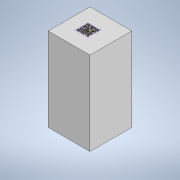
# Autodesk Inventor part: OBJECT
Saved by Autodesk Inventor 2022.2 (Build 262287000, 287)
## iProperties
Created: 2022-02-23
Part Number: OBJECT
Material: Generic
Document SubType Name: Modeling
Designer: ONG
Density: 1 g/cm^3
Appearance: Default
Author: ONG
Autodesk Inventor part; units mm, degrees
ref_plane "YZ Plane" through (0, 0, 0) normal (1, 0, 0) x (0, 1, 0)
ref_plane "XZ Plane" through (0, 0, 0) normal (0, 1, 0) x (-1, 0, 0)
ref_plane "XY Plane" through (0, 0, 0) normal (0, 0, 1) x (1, 0, 0)
sketch "Sketch1" plane through (0, 0, 0) normal (0, 1, 0) x (-1, 0, 0)
  line L0 (-50, -50) -> (50, -50)
  line L1 (50, -50) -> (50, 50)
  line L2 (50, 50) -> (-50, 50)
  line L3 (-50, 50) -> (-50, -50)
  line L4 (-50, -50) -> (50, 50) construction
  line L5 (50, -50) -> (-50, 50) construction
  point P0 (0, 0)
  dimension "d0" = 100
  dimension "d1" = 100
  constraints: 12 end point, 2 midpoint, 2 parallel, 1 horizontal, 1 perpendicular
  measures "d0" distance of L2.end L1.end
  measures "d1" distance of L1.end L0.end
extrude "Extrusion1" add sketch "Sketch1" along normal blind 200
sketch "Sketch3" plane through (50, 0, -50) normal (0, 0, -1) x (-1, 0, 0)
  line L0 (21.1023, 115.1057) -> (65.8801, 115.1057) construction
  line L1 (65.8801, 115.1057) -> (65.8801, 70.3279) construction
  line L2 (65.8801, 70.3279) -> (21.1023, 70.3279) construction
  line L3 (21.1023, 70.3279) -> (21.1023, 115.1057) construction
  point P0 (50, 0)
  constraints: 2 other
sketch "Sketch4" plane through (0, 200, 0) normal (0, 1, 0) x (1, 0, 0)
  line L0 (-19.649, 14.8569) -> (11.1811, 14.8569) construction
  line L1 (11.1811, 14.8569) -> (11.1811, -15.9732) construction
  line L2 (11.1811, -15.9732) -> (-19.649, -15.9732) construction
  line L3 (-19.649, -15.9732) -> (-19.649, 14.8569) construction
  point P0 (0, 0)
  constraints: 2 other
sketch "Sketch5" plane through (0, 0, 0) normal (0, -1, 0) x (1, 0, 0)
  line L0 (-15.5915, 13.2858) -> (16.9921, 13.2858) construction
  line L1 (16.9921, 13.2858) -> (16.9921, -19.2978) construction
  line L2 (16.9921, -19.2978) -> (-15.5915, -19.2978) construction
  line L3 (-15.5915, -19.2978) -> (-15.5915, 13.2858) construction
  point P0 (0, 0)
  constraints: 2 other
body "Solid1"
